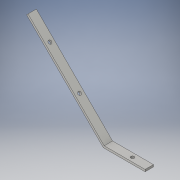
# Autodesk Inventor part: ChassisClamp
Saved by Autodesk Inventor 2016 (Build 200138000, 138)
## iProperties
Created: 2017-04-26
Part Number: ChassisClamp
Material: Generic
Document SubType Name: Modeling
Designer: Evan Phil George
Density: 1 g/cm^3
Appearance: Default
Author: Evan Phil George
Autodesk Inventor part; units mm, degrees
ref_plane "YZ Plane" through (0, 0, 0) normal (1, 0, 0) x (0, 1, 0)
ref_plane "XZ Plane" through (0, 0, 0) normal (0, 1, 0) x (-1, 0, 0)
ref_plane "XY Plane" through (0, 0, 0) normal (0, 0, 1) x (1, 0, 0)
sketch "Sketch1" plane through (0, 0, 0) normal (0, 0, 1) x (1, 0, 0)
  line L0 (0, 0) -> (50, 0)
  line L1 (0, 0) -> (-91.9239, 91.9239)
  line L2 (0, 0) -> (130, 0) construction
  line L3 (-91.9239, 91.9239) -> (-90.1561, 93.6916)
  line L4 (-91.9239, 91.9239) -> (-89.4239, 91.9239) construction
  line L5 (-90.1561, 93.6916) -> (1.0355, 2.5)
  line L6 (50, 0) -> (50, 2.5)
  line L7 (50, 2.5) -> (1.0355, 2.5)
  dimension "d0" = 50
  dimension "d1" = 130
  dimension "d2" = 135
  dimension "d3" = 2.5
  dimension "d4" = 45
  dimension "d5" = 90
  dimension "d6" = 2.5
  constraints: 16 end point, 3 horizontal, 2 equal length, 1 perpendicular, 1 vertical
  measures "d0" distance of L0.start L0.end
  measures "d1" distance of L0.start L1.end
  measures "d2" angle of L2 L1
  measures "d3" distance of L1.end L3.end
  measures "d4" angle of L4 L3
  measures "d5" angle of L3 L5
  measures "d6" distance of L0.end L6.end
extrude "Extrusion1" add sketch "Sketch1" along normal blind 10
sketch "Sketch2" plane through (0, 0, 0) normal (0, -1, 0) x (1, 0, 0)
  line L0 (0, 0) -> (0, 10) projected
  line L1 (0, 5) -> (30, 5)
  circle A0 centre (30, 5) radius 2
  dimension "d9" = 30
  dimension "d10" = 4
  constraints: 2 end point, 1 centre point, 1 coincident, 1 horizontal, 1 midpoint
  measures "d9" distance of L1.start L1.end
  measures "d10" diameter of A0
extrude "Extrusion2" cut sketch "Sketch2" against normal blind 10
sketch "Sketch3" plane through (0, 0, 10) normal (-0.7071, -0.7071, 0) x (-0.7071, 0.7071, 0)
  line L0 (0, 10) -> (0, 0) projected
  line L1 (0, 5) -> (50, 5)
  line L2 (0, 5) -> (50, 5) construction
  line L3 (50, 5) -> (100, 5)
  line L4 (50, 5) -> (100, 5) construction
  circle A0 centre (100, 5) radius 2
  circle A1 centre (50, 5) radius 2
  dimension "d13" = 50
  dimension "d14" = 0
  dimension "d15" = 50
  dimension "d16" = 0
  dimension "d17" = 4
  dimension "d18" = 4
  constraints: 8 end point, 3 collinear, 3 horizontal, 2 centre point, 2 coincident, 1 midpoint
  measures "d13" distance of L1.start L1.end
  measures "d14" distance between parallel lines of L1 L2
  measures "d15" distance of L2.end L3.end
  measures "d16" distance between parallel lines of L3 L4
  measures "d17" diameter of A0
  measures "d18" diameter of A1
extrude "Extrusion3" cut sketch "Sketch3" against normal blind 10
body "Solid1"
